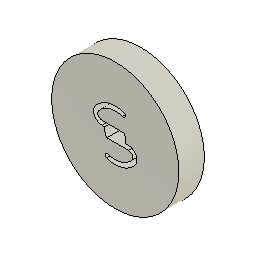
Wheel (Autodesk Fusion 360 design; units mm, degrees)
Autodesk Fusion 360 part; units mm, degrees
note: some values were not read from the file. Set by a fixed rule: which sketch regions a step uses.
sketch "Sketch1" plane through (0, 0, 0) normal (0, 1, 0) x (1, 0, 0)
  arc A0 (2, -1.5) -> (2.5, 0) centre (0, 0) ccw
  arc A1 (-2.5, 0) -> (-2.4495, -0.5) centre (0, 0) ccw
  line L0 (-3.1225, -0.5) -> (-2.4495, -0.5)
  line L1 (-3.1225, -1.5) -> (2, -1.5)
  arc A2 (-3.9031, -3.125) -> (1.7101, -4.6985) centre (0, 0) ccw
  arc A3 (-4.6837, -3.75) -> (2.0521, -5.6382) centre (0, 0) ccw
  arc A4 (-15, 0) -> (15, 0) centre (0, 0) ccw
  arc A5 (2.0521, -5.6382) -> (1.7101, -4.6985) centre (1.8811, -5.1683) ccw
  arc A6 (-3.1225, -1.5) -> (-3.9031, -3.125) centre (-3.1225, -2.5) ccw
  arc A7 (-3.1225, -0.5) -> (-4.6837, -3.75) centre (-3.1225, -2.5) ccw
  arc A8 (15, 0) -> (-15, 0) centre (0, 0) ccw
  arc A9 (4.6837, 3.75) -> (-2.0521, 5.6382) centre (0, 0) ccw
  arc A10 (-2.0521, 5.6382) -> (-1.7101, 4.6985) centre (-1.8811, 5.1683) ccw
  arc A11 (3.1225, 0.5) -> (4.6837, 3.75) centre (3.1225, 2.5) ccw
  arc A12 (3.1225, 1.5) -> (3.9031, 3.125) centre (3.1225, 2.5) ccw
  arc A13 (2.5, 0) -> (2.4495, 0.5) centre (0, 0) ccw
  arc A14 (3.9031, 3.125) -> (-1.7101, 4.6985) centre (0, 0) ccw
  arc A15 (-2, 1.5) -> (-2.5, 0) centre (0, 0) ccw
  line L2 (3.1225, 1.5) -> (-2, 1.5)
  line L3 (3.1225, 0.5) -> (2.4495, 0.5)
  dimension "d9" = 2.5
  dimension "d10" = 5
  dimension "d11" = 6
  dimension "d15" = 1
  dimension "d19" = 15
  dimension "d21" = 360
  measures "d9" radius of A0
  measures "d10" radius of A2
  measures "d11" radius of A3
  measures "d15" distance of L0 L1
  measures "d19" radius of A4
extrude "Extrude1" add sketch "Sketch1" along normal mid plane 6
